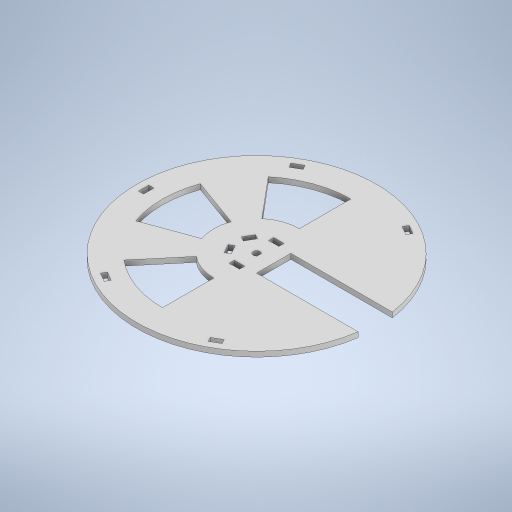
# Autodesk Inventor part: rolling_plate
Saved by Autodesk Inventor 2024 (Build 280153000, 153)
## iProperties
Created: 2024-04-09
Part Number: rolling_plate
Material: 一般
Document SubType Name: Modeling
Designer: USER
Density: 1 g/cm^3
Appearance: 預設
Author: USER
Autodesk Inventor part; units mm, degrees
ref_plane "YZ Plane" through (0, 0, 0) normal (1, 0, 0) x (0, 1, 0)
ref_plane "XZ Plane" through (0, 0, 0) normal (0, 1, 0) x (-1, 0, 0)
ref_plane "XY Plane" through (0, 0, 0) normal (0, 0, 1) x (1, 0, 0)
sketch "草圖1" plane through (0, 0, 0) normal (0, 1, 0) x (-1, 0, 0)
  circle A0 centre (0, 0) radius 70
  circle A1 centre (0, 0) radius 25
  line L0 (-70, 10) -> (-10, 10)
  line L1 (-10, 10) -> (-10, -10)
  line L2 (-10, -10) -> (-70, -10)
  line L3 (-70, -10) -> (-70, 10)
  line L4 (0, 0) -> (0, -55)
  line L5 (0, 0) -> (35.3533, -42.1324)
  arc A2 (0, -55) -> (35.3533, -42.1324) centre (0, 0) ccw
  line L6 (0, 0) -> (51.6831, -18.8111)
  line L7 (0, 0) -> (51.6831, 18.8111)
  arc A3 (51.6831, -18.8111) -> (51.6831, 18.8111) centre (0, 0) ccw
  line L8 (0, 0) -> (35.3533, 42.1324)
  line L9 (0, 0) -> (0, 55)
  arc A4 (35.3533, 42.1324) -> (0, 55) centre (0, 0) ccw
  line L10 (-9.3, -13.3795) -> (-36.7, -13.3795)
  line L11 (-36.7, -13.3795) -> (-36.7, -69.3795)
  line L12 (-36.7, -69.3795) -> (-9.3, -69.3795)
  line L13 (-9.3, -69.3795) -> (-9.3, -13.3795)
  line L14 (-7.8, -20.3795) -> (-10.8, -20.3795)
  line L15 (-10.8, -20.3795) -> (-10.8, -27.3795)
  line L16 (-10.8, -27.3795) -> (-7.8, -27.3795)
  line L17 (-7.8, -27.3795) -> (-7.8, -20.3795)
  line L18 (-7.8, -55.3795) -> (-10.8, -55.3795)
  line L19 (-10.8, -55.3795) -> (-10.8, -62.3795)
  line L20 (-10.8, -62.3795) -> (-7.8, -62.3795)
  line L21 (-7.8, -62.3795) -> (-7.8, -55.3795)
  line L22 (-35.2, -20.3795) -> (-38.2, -20.3795)
  line L23 (-38.2, -20.3795) -> (-38.2, -27.3795)
  line L24 (-38.2, -27.3795) -> (-35.2, -27.3795)
  line L25 (-35.2, -27.3795) -> (-35.2, -20.3795)
  line L26 (-35.2, -48.3795) -> (-38.2, -48.3795)
  line L27 (-38.2, -48.3795) -> (-38.2, -55.3795)
  line L28 (-38.2, -55.3795) -> (-35.2, -55.3795)
  line L29 (-35.2, -55.3795) -> (-35.2, -48.3795)
  circle A5 centre (0, 0) radius 2
  line L30 (-1.5, 1.3229) -> (-1.5, -1.3229)
  point P0 (-23, -13.3795)
  point P1 (-9.3, -20.3795)
  point P2 (-9.3, -62.3795)
  point P3 (-36.7, -20.3795)
  point P4 (-36.7, -48.3795)
  point P5 (16.0697, -19.1511)
  point P6 (0, -25)
  point P7 (-69.282, 10)
  point P8 (-69.282, -10)
  point P9 (16.0697, 19.1511)
  point P10 (0, 25)
  point P11 (23.4923, -8.5505)
  point P12 (23.4923, 8.5505)
  point P13 (-70, 0)
  dimension "d0" = 140
  dimension "d1" = 50
  dimension "d2" = 20
  dimension "d3" = 60
  dimension "d4" = 55
  dimension "d5" = 40
  dimension "d6" = 55
  dimension "d9" = 140
  dimension "d11" = 13
  dimension "d12" = 27.4
  dimension "d13" = 56
  dimension "d14" = 7
  dimension "d15" = 3
  dimension "d16" = 7
  dimension "d17" = 7
  dimension "d18" = 3
  dimension "d19" = 7
  dimension "d20" = 7
  dimension "d21" = 3
  dimension "d22" = 7
  dimension "d23" = 7
  dimension "d24" = 3
  dimension "d25" = 21
  dimension "d28" = 4
  dimension "d29" = 1.5
  constraints: 62 end point, 12 parallel, 10 point on circle, 6 centre point, 6 coincident, 6 horizontal, 6 midpoint, 6 perpendicular, 6 point on line, 2 vertical, 1 horizontal alignment, 1 vertical alignment, 17 other
  measures "d0" diameter of A0
  measures "d1" diameter of A1
  measures "d2" distance of L2.end L0.start
  measures "d3" distance of L1.end L2.end
  measures "d4" distance of L4.start L4.end
  measures "d5" angle of L4 L5
  measures "d6" distance of L4.start L5.end
  measures "d11" horizontal distance of L1.end point (-23, -13.379)
  measures "d12" distance of L11.end L12.end
  measures "d13" distance of L12.end L10.start
  measures "d14" distance of L16.end L14.start
  measures "d15" distance of L15.end L16.end
  measures "d16" distance from line of L10.start L14
  measures "d17" distance of L20.end L18.start
  measures "d18" distance of L19.end L20.end
  measures "d19" distance from line of L12.end L20
  measures "d20" distance of L24.end L22.start
  measures "d21" distance of L23.end L24.end
  measures "d22" vertical distance of L10.end L22.start
  measures "d23" distance of L28.end L26.start
  measures "d24" distance of L27.end L28.end
  measures "d25" distance of L24.end L26.start
  measures "d28" diameter of A5
  measures "d29" distance between parallel lines of L4 L30
extrude "擠出1" add sketch "草圖1" along normal blind 3 contours L13 L20 L21 L18 L16 L17 A1 L4 A2 L5 L6 A3 L7 L8 A4 L9 L0 A0 | A0 L11 L28 L29 L26 L24 L25 L22 L10 A1 L15 L16 L13 L18 L19 L20 | A0 L2 A1 L10 L11 L22 L23 L24 L26 L27 L28 | L20 L19 L18 L13 | L13 L18 L21 L20 | L28 L27 L26 L11 | L11 L26 L29 L28 | A1 L9 A5 L4 L17 L14 L13 L10 L2 L1 L0 | L16 L15 A1 L13 | L13 A1 L17 L16 | A1 L8 A5 L9 | L10 L13 L14 L15 A1 | L24 L23 L22 L11 | L11 L22 L25 L24 | L13 L14 L17 A1 | A1 L15 L14 L13 | A1 L7 A5 L8 | A1 L6 A5 L7 | L30 A5 | L4 A5 L5 A1 | A5 L6 A1 L5
sketch "草圖2" plane through (0, 3, 0) normal (0, 1, 0) x (1, 0, 0)
  line L0 (-66, 3) -> (-63, 3)
  line L1 (-63, 3) -> (-63, -3)
  line L2 (-63, -3) -> (-66, -3)
  line L3 (-66, -3) -> (-66, 3)
  line L4 (-35.5981, -55.6577) -> (-34.0981, -53.0596)
  line L5 (-34.0981, -53.0596) -> (-28.9019, -56.0596)
  line L6 (-28.9019, -56.0596) -> (-30.4019, -58.6577)
  line L7 (-30.4019, -58.6577) -> (-35.5981, -55.6577)
  line L8 (30.4019, -58.6577) -> (28.9019, -56.0596)
  line L9 (28.9019, -56.0596) -> (34.0981, -53.0596)
  line L10 (34.0981, -53.0596) -> (35.5981, -55.6577)
  line L11 (35.5981, -55.6577) -> (30.4019, -58.6577)
  line L12 (66, -3) -> (63, -3)
  line L13 (63, -3) -> (63, 3)
  line L14 (63, 3) -> (66, 3)
  line L15 (66, 3) -> (66, -3)
  line L16 (35.5981, 55.6577) -> (34.0981, 53.0596)
  line L17 (34.0981, 53.0596) -> (28.9019, 56.0596)
  line L18 (28.9019, 56.0596) -> (30.4019, 58.6577)
  line L19 (30.4019, 58.6577) -> (35.5981, 55.6577)
  line L20 (-30.4019, 58.6577) -> (-28.9019, 56.0596)
  line L21 (-28.9019, 56.0596) -> (-34.0981, 53.0596)
  line L22 (-34.0981, 53.0596) -> (-35.5981, 55.6577)
  line L23 (-35.5981, 55.6577) -> (-30.4019, 58.6577)
  point P0 (0, 0)
  point P1 (-63, 0)
  point P2 (-31.5, -54.5596)
  point P3 (31.5, -54.5596)
  point P4 (63, 0)
  point P5 (31.5, 54.5596)
  point P6 (-31.5, 54.5596)
  dimension "d30" = 3
  dimension "d31" = 6
  dimension "d32" = 63
  dimension "d37" = 360
  constraints: 48 end point, 2 parallel, 1 horizontal, 1 horizontal alignment, 1 midpoint, 1 perpendicular, 55 other
  measures "d30" distance of L1.end L2.end
  measures "d31" distance of L2.end L0.start
  measures "d32" distance from line of point (0, 0) L1
extrude "擠出2" cut sketch "草圖2" against normal through all contours L0 L1 L2 L3 | L4 L5 L6 L7 | L8 L9 L10 L11 | L16 L17 L18 L19 | L20 L21 L22 L23
sketch "草圖3" plane through (0, 3, 0) normal (0, 1, 0) x (1, 0, 0)
  line L0 (-3, 13) -> (3, 13)
  line L1 (3, 13) -> (3, 10)
  line L2 (3, 10) -> (-3, 10)
  line L3 (-3, 10) -> (-3, 13)
  line L4 (-12.7583, 3.9019) -> (-9.7583, 9.0981)
  line L5 (-9.7583, 9.0981) -> (-7.1603, 7.5981)
  line L6 (-7.1603, 7.5981) -> (-10.1603, 2.4019)
  line L7 (-10.1603, 2.4019) -> (-12.7583, 3.9019)
  line L8 (-9.7583, -9.0981) -> (-12.7583, -3.9019)
  line L9 (-12.7583, -3.9019) -> (-10.1603, -2.4019)
  line L10 (-10.1603, -2.4019) -> (-7.1603, -7.5981)
  line L11 (-7.1603, -7.5981) -> (-9.7583, -9.0981)
  line L12 (3, -13) -> (-3, -13)
  line L13 (-3, -13) -> (-3, -10)
  line L14 (-3, -10) -> (3, -10)
  line L15 (3, -10) -> (3, -13)
  point P0 (0, 0)
  point P1 (0, 10)
  point P2 (-8.6603, 5)
  point P3 (-8.6603, -5)
  point P4 (0, -10)
  dimension "d39" = 6
  dimension "d40" = 3
  dimension "d41" = 10
  dimension "d44" = 180
  constraints: 32 end point, 2 parallel, 1 horizontal, 1 midpoint, 1 perpendicular, 1 vertical alignment, 28 other
  measures "d39" distance of L1.end L2.end
  measures "d40" distance of L0.end L1.end
  measures "d41" distance from line of point (0, 0) L2
extrude "擠出3" cut sketch "草圖3" against normal through all
